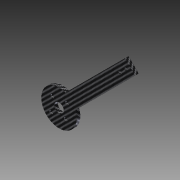
# Autodesk Inventor part: arm
Saved by Autodesk Inventor 2015 (Build 190159000, 159)
## iProperties
Created: 2016-11-27
Part Number: arm
Material: Generic
Document SubType Name: Modeling
Designer: Hampus
Density: 1 g/cm^3
Appearance: Carbon Fiber
Author: Hampus
Autodesk Inventor part; units mm, degrees
ref_plane "YZ Plane" through (0, 0, 0) normal (1, 0, 0) x (0, 1, 0)
ref_plane "XZ Plane" through (0, 0, 0) normal (0, 1, 0) x (-1, 0, 0)
ref_plane "XY Plane" through (0, 0, 0) normal (0, 0, 1) x (1, 0, 0)
sketch "Sketch1" plane through (0, 0, 0) normal (0, 1, 0) x (-1, 0, 0)
  circle A0 centre (4.364, -12.8492) radius 1.25
  line L0 (2.1213, -19.0919) -> (-8.4853, -8.4853)
  line L1 (10.6066, -10.6066) -> (0, 0)
  line L2 (0, 0) -> (-8.4853, -8.4853)
  circle A1 centre (-0.7071, -7.7782) radius 1.25
  line L3 (2.1213, -19.0919) -> (41.8977, -58.8682)
  line L4 (10.6066, -10.6066) -> (50.383, -50.383)
  arc A2 (41.8977, -58.8682) -> (50.383, -50.383) centre (55.8614, -64.3467) ccw
  circle A3 centre (62.579, -71.0642) radius 1.5
  circle A4 centre (49.1439, -57.6292) radius 1.5
  circle A5 centre (50.2046, -70.0036) radius 1.5
  circle A6 centre (61.5183, -58.6899) radius 1.5
  point P0 (0, 0)
  dimension "d3" = 3
  dimension "d4" = 3
  dimension "d5" = 3
  dimension "d6" = 3
  constraints: 10 end point, 7 centre point, 2 point on circle
  measures "d3" diameter of A3
  measures "d4" diameter of A4
  measures "d5" diameter of A5
  measures "d6" diameter of A6
extrude "Extrusion1" add sketch "Sketch1" along normal blind 3
sketch "Sketch2" plane through (0, 3, 0) normal (0, 1, 0) x (1, 0, 0)
  arc A0 (-41.8977, 58.8682) -> (-50.383, 50.383) centre (-55.8614, 64.3467) ccw projected
  circle A1 centre (-55.8614, 64.3467) radius 4
  point P0 (0, 0)
  dimension "d9" = 8
  constraints: 1 centre point, 1 coincident
  measures "d9" diameter of A1
extrude "Extrusion2" cut sketch "Sketch2" against normal blind 3
body "Solid1"
